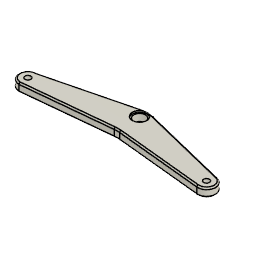
RV1-SUS-001_Rocker_Differential_Arm (Autodesk Fusion 360 design; units mm, degrees)
part number: 2026-02-10-00-22-16-787
Autodesk Fusion 360 part; units mm, degrees
sketch "Sketch1" plane through (0, 0, 0) normal (0, 0, 1) x (1, 0, 0)
  line L0 (0, 0) -> (254, 0) construction
  line L1 (0, 0) -> (-254, 0) construction
  circle A0 centre (-254, 0) radius 8.128
  circle A1 centre (254, 0) radius 8.128
  line L2 (0, 0) -> (0, 63.5) construction
  circle A2 centre (0, 63.5) radius 16.5
  line L3 (-254, -25.4) -> (0, 0)
  line L4 (0, 0) -> (251.46, -25.2727)
  arc A3 (-254, 25.4) -> (-248.9703, -24.897) centre (-254, 0) ccw
  arc A4 (251.46, -25.2727) -> (258.9348, 24.916) centre (254, 0) ccw
  line L5 (-0.0285, 88.9) -> (-254, 25.4)
  line L6 (-0.0285, 88.9) -> (258.9348, 24.916)
  arc A5 (11.8546, 85.9639) -> (-11.9289, 85.9245) centre (0, 63.5) ccw
  dimension "d1" = 254
  dimension "d2" = 254
  dimension "d3" = 16.256
  dimension "d4" = 16.256
  dimension "d5" = 33
  constraint coincident L0.start L1.start
  constraint horizontal L0
  constraint parallel L0 L1
  constraint coincident L1.end A0.centre
  constraint coincident L0.end A1.centre
  constraint concentric A0 A3
  constraint concentric A1 A4
  constraint perpendicular L0 L2
  constraint coincident L2.end A2.centre
  constraint coincident L3.start A3
  constraint tangent L4 A4
  constraint coincident L3 A3.end
  constraint concentric A2 A5
  constraint coincident L5.start A5
  constraint coincident L6 A5.start
  constraint coincident L5 A5.end
  measures "d1" distance of L0.start L0.end
  measures "d2" distance of L0.start L1.end
  measures "d3" diameter of A0
  measures "d4" diameter of A1
  measures "d5" diameter of A2
extrude "Extrude1" add sketch "Sketch1" along normal blind 24.2 contours L3 L4 A3 A4 L5 L6
fillet "Fillet1" radius 76.2 2 edges at (0, 0, 12.1) (-0.0285, 88.9, 12.1)
fillet "Fillet2" radius 3.81 16 edges at (-130.8006, -13.0801, 24.2) (-0.0001, -0.382, 24.2) (129.5305, -13.0183, 24.2) (279.1229, -3.7416, 24.2) (-279.4, 0, 24.2) (-130.8006, -13.0801, 0) (-0.0001, -0.382, 0) (129.5305, -13.0183, 0) (279.1229, -3.7416, 0) (-279.4, 0, 0) (138.6465, 54.6365, 24.2) (-0.0253, 86.5815, 24.2) (-136.2013, 54.853, 24.2) (-136.2013, 54.853, 0) (-0.0253, 86.5815, 0) (138.6465, 54.6365, 0)
scale "Scale1" factor 0.5 about (-16.5, 63.5, 24.2) bodies 1
sketch "Sketch2" plane through (0, 0, 24.2) normal (0, 0, 1) x (-1, 0, 0)
  circle A0 centre (8.25, -63.5) radius 8.25
  circle A1 centre (-118.75, -31.75) radius 4.064
  circle A2 centre (135.25, -31.75) radius 4.064
  line L0 (135.3412, -20.9554) -> (12.2402, -33.2655)
  arc A3 (4.259, -33.2635) -> (12.2402, -33.2655) centre (8.2595, 6.541) ccw
  line L1 (4.259, -33.2635) -> (-117.6705, -21.0091)
  arc A4 (-117.6705, -21.0091) -> (-120.8054, -42.3475) centre (-118.75, -31.75) ccw
  line L2 (-120.8054, -42.3475) -> (-0.4722, -72.0791)
  arc A5 (-0.4722, -72.0791) -> (16.9892, -72.0549) centre (8.2097, -36.9408) ccw
  line L3 (16.9892, -72.0549) -> (135.0248, -42.5427)
  arc A6 (135.0248, -42.5427) -> (135.3412, -20.9554) centre (135.25, -31.75) ccw
  circle A7 centre (8.25, -63.5) radius 10.25
  dimension "d13" = 20.5
  constraint concentric A0 A7
  measures "d13" diameter of A7
extrude "Extrude2" cut sketch "Sketch2" against normal blind 2.1 contours A5 A7 | A5 A7
